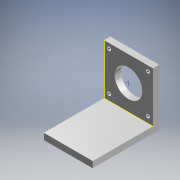
# Autodesk Inventor part: head-baseblate
Saved by Autodesk Inventor 2016 (Build 200138000, 138)
## iProperties
Created: 2015-04-29
Part Number: head-baseblate
Material: Aluminum 6061
Document SubType Name: Modeling
Designer: ax
Density: 2.7 g/cm^3
Appearance: Aluminum - Flat
Mass: 43.451 g
Surface Area: 82.9126 cm^2
Volume: 16.093 cm^3
Author: ax
Autodesk Inventor part; units mm, degrees
ref_plane "YZ Plane" through (0, 0, 0) normal (1, 0, 0) x (0, 1, 0)
ref_plane "XZ Plane" through (0, 0, 0) normal (0, 1, 0) x (-1, 0, 0)
ref_plane "XY Plane" through (0, 0, 0) normal (0, 0, 1) x (1, 0, 0)
sketch "Sketch1" plane through (0, 0, 0) normal (0, 0, 1) x (1, 0, 0)
  line L0 (0, 0) -> (39, 0)
  line L1 (39, 0) -> (39, -53)
  line L2 (39, -53) -> (0, -53)
  line L3 (0, -53) -> (0, 0)
  dimension "d0" = 39
  dimension "d1" = 53
  constraints: 8 end point, 2 parallel, 1 horizontal, 1 perpendicular
  measures "d0" distance of L1.end L2.end
  measures "d1" distance of L0.end L1.end
extrude "Extrusion1" add sketch "Sketch1" along normal blind 5
sketch "Sketch2" plane through (0, 0, 5) normal (0, 0, 1) x (1, 0, 0)
  line L0 (39, 0) -> (0, 0) projected
  line L1 (39, -53) -> (39, 0) projected
  line L2 (0, 0) -> (39, 0)
  line L3 (39, 0) -> (39, -5)
  line L4 (39, -5) -> (0, -5)
  line L5 (0, -5) -> (0, 0)
  dimension "d4" = 5
  constraints: 8 end point, 2 parallel, 1 horizontal, 1 perpendicular, 1 point on line
  measures "d4" distance of L2.end L3.end
extrude "Extrusion2" add sketch "Sketch2" along normal blind 40
sketch "Sketch3" plane through (0, -5, 5) normal (0, -1, 0) x (1, 0, 0)
  line L0 (0, 0) -> (0, 40) projected
  line L1 (0, 0) -> (39, 0) projected
  point P0 (0, -5)
  point P1 (19.5, 20)
  point P2 (4, 5)
  point P3 (4, 36)
  point P4 (35, 5)
  point P5 (35, 36)
  dimension "d7" = 19.5
  dimension "d8" = 20
  dimension "d9" = 5
  dimension "d10" = 4
  dimension "d13" = 31
  dimension "d16" = 31
  constraints: 1 horizontal, 1 vertical, 3 other
  measures "d7" distance from line of L0 point (19.5, 20)
  measures "d8" distance from line of L1 point (19.5, 20)
  measures "d9" distance from line of L1 point (4, 5)
  measures "d10" distance from line of L0 point (4, 5)
  measures "d13" distance of point (4, 5) point (4, 36)
  measures "d16" distance of point (4, 5) point (35, 5)
hole "Hole1" at (19.5, -5, 25) direction (0, 1, 0) diameter 22 end through all
hole "Hole2" at (4, -5, 10) at (4, -5, 41) at (35, -5, 41) at (35, -5, 10) direction (0, 1, 0) diameter 3 end through all
body "Solid1"
